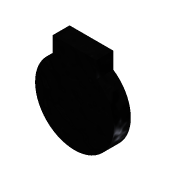
# Autodesk Inventor part: Encoder model
Saved by Autodesk Inventor 2016 (Build 200138000, 138)
## iProperties
Created: 2015-05-19
Part Number: Encoder model
Material: Generic
Document SubType Name: Modeling
Designer: Andy
Density: 1 g/cm^3
Appearance: Default
Mass: 33.0024 g
Surface Area: 80.1106 cm^2
Volume: 33.0024 cm^3
Author: Andy
Autodesk Inventor part; units mm, degrees
ref_plane "YZ Plane" through (0, 0, 0) normal (1, 0, 0) x (0, 1, 0)
ref_plane "XZ Plane" through (0, 0, 0) normal (0, 1, 0) x (-1, 0, 0)
ref_plane "XY Plane" through (0, 0, 0) normal (0, 0, 1) x (1, 0, 0)
sketch "Sketch1" plane through (0, 0, 0) normal (0, 1, 0) x (-1, 0, 0)
  circle A0 centre (0, 0) radius 28
  dimension "d0" = 56
  constraints: 1 centre point, 1 coincident
  measures "d0" diameter of A0
extrude "Extrusion1" add sketch "Sketch1" along normal blind 12
sketch "Sketch3" plane through (0, 0, 0) normal (0, 0, 1) x (1, 0, 0)
  line L0 (0, 11.8294) -> (-15.4991, 12)
  line L1 (28, 12) -> (-28, 12) projected
  line L2 (-15.4991, 12) -> (-15.4991, -22.0673)
  line L3 (-28, 0) -> (28, 0) projected
  line L4 (-15.4991, 12) -> (15.5009, 12)
  line L5 (15.5009, 12) -> (15.5009, 0)
  line L6 (15.5009, 0) -> (-15.4991, 0)
  line L7 (-15.4991, 0) -> (-15.4991, 12)
  point P0 (0, 0)
  dimension "d5" = 15.5
  dimension "d6" = 31
  constraints: 12 end point, 2 parallel, 2 perpendicular, 2 point on line, 1 horizontal
  measures "d5" distance of L0.start L0.end
  measures "d6" distance of L5.end L6.end
extrude "Extrusion2" add sketch "Sketch3" along normal blind 35
sketch "Sketch4" plane through (0, 12, 0) normal (0, 1, 0) x (1, 0, 0)
  arc A0 (15.5009, -23.3178) -> (-15.4991, -23.3191) centre (0, 0) ccw projected
  circle A1 centre (0, 0) radius 3
  dimension "d9" = 6
  constraints: 1 centre point, 1 coincident
  measures "d9" diameter of A1
extrude "Extrusion3" add sketch "Sketch4" along normal blind 10
body "Solid1"
